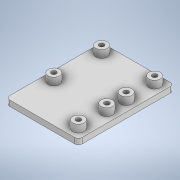
# Autodesk Inventor part: adc_board_rack
Saved by Autodesk Inventor 2022 (Build 260153000, 153)
## iProperties
Created: 2021-09-06
Part Number: adc_board_rack
Material: Generic
Document SubType Name: Modeling
Designer: dsdan
Density: 1 g/cm^3
Appearance: Default
Author: dsdan
Autodesk Inventor part; units mm, degrees
ref_plane "YZ Plane" through (0, 0, 0) normal (1, 0, 0) x (0, 1, 0)
ref_plane "XZ Plane" through (0, 0, 0) normal (0, 1, 0) x (-1, 0, 0)
ref_plane "XY Plane" through (0, 0, 0) normal (0, 0, 1) x (1, 0, 0)
sketch "Sketch1" plane through (0, 0, 0) normal (0, 1, 0) x (-1, 0, 0)
  line L0 (0, 0) -> (38.2, 0)
  line L1 (38.2, 0) -> (38.2, -25.2)
  line L2 (38.2, -25.2) -> (0, -25.2)
  line L3 (0, -25.2) -> (0, 0)
  circle A0 centre (33.1, -20.1) radius 1.3
  circle A1 centre (5.1, -5.1) radius 1.3
  circle A2 centre (5.1, -20.1) radius 1.3
  line L4 (0, 0) -> (38.2, -25.2) construction
  line L5 (38.2, 0) -> (0, -25.2) construction
  line L6 (5.1, -5.1) -> (33.1, -20.1) construction
  point P0 (19.1, -12.6)
  dimension "d1" = 15
  dimension "d2" = 28
  dimension "d3" = 2.6
  dimension "d4" = 2.6
  dimension "d5" = 2.6
  dimension "d18" = 25.2
  dimension "d19" = 38.2
  constraints: 14 end point, 3 centre point, 2 midpoint, 2 parallel, 1 horizontal, 1 horizontal alignment, 1 perpendicular, 1 vertical alignment
  measures "d1" distance of A2.centre L6.start
  measures "d2" distance of L6.end A2.centre
  measures "d3" diameter of A0
  measures "d4" diameter of A2
  measures "d5" diameter of A1
  measures "d18" distance of L0.end L1.end
  measures "d19" distance of L1.end L2.end
extrude "Extrusion1" add sketch "Sketch1" along normal blind 3
sketch "Sketch2" plane through (0, 3, 0) normal (0, 1, 0) x (1, 0, 0)
  circle A0 centre (-5.1, 5.1) radius 1.3 projected
  circle A1 centre (-5.1, 5.1) radius 3
  circle A2 centre (-5.1, 20.1) radius 1.3 projected
  circle A3 centre (-5.1, 20.1) radius 3
  circle A4 centre (-33.1, 20.1) radius 1.3 projected
  circle A5 centre (-33.1, 20.1) radius 3
  point P0 (0, 0)
  dimension "d12" = 6
  dimension "d13" = 6
  dimension "d14" = 6
  constraints: 3 centre point, 3 coincident
  measures "d12" diameter of A5
  measures "d13" diameter of A1
  measures "d14" diameter of A3
extrude "Extrusion2" add sketch "Sketch2" along normal blind 4
pattern_linear "Rectangular Pattern1" count 2 spacing 25.2 along (0, 0, 1) of "Extrusion1", "Extrusion2"
fillet "Fillet2" radius 2 4 edges at (0, 1.5, 25.2) (0, 1.5, -25.2) (-38.2, 1.5, -25.2) (-38.2, 1.5, 25.2)
equation "\"d4\" = d3"
equation "\"d5\" = d3"
equation "\"d13\" = d12"
equation "\"d14\" = d12"
equation "\"d7\" = d8"
equation "\"d8\" = 3"
body "Solid1"
